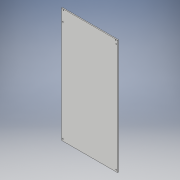
# Autodesk Inventor part: GlyphPlateUnderside
Saved by Autodesk Inventor 2017 (Build 210142000, 142)
## iProperties
Created: 2018-01-27
Part Number: GlyphPlateUnderside
Material: Generic
Document SubType Name: Modeling
Designer: User
Density: 1 g/cm^3
Appearance: Default
Author: User
Autodesk Inventor part; units mm, degrees
ref_plane "YZ Plane" through (0, 0, 0) normal (1, 0, 0) x (0, 1, 0)
ref_plane "XZ Plane" through (0, 0, 0) normal (0, 1, 0) x (-1, 0, 0)
ref_plane "XY Plane" through (0, 0, 0) normal (0, 0, 1) x (1, 0, 0)
sketch "Sketch1" plane through (0, 0, 0) normal (0, 0, 1) x (1, 0, 0)
  line L0 (0, 0) -> (185.8518, 0)
  line L1 (185.8518, 0) -> (185.8518, 381)
  line L2 (185.8518, 381) -> (0, 381)
  line L3 (0, 381) -> (0, 0)
  dimension "d0" = 185.8518
  dimension "d1" = 381
  constraints: 8 end point, 2 parallel, 1 horizontal, 1 perpendicular
  measures "d0" distance of L2.end L1.end
  measures "d1" distance of L1.end L0.end
extrude "Extrusion1" add sketch "Sketch1" along normal blind 3.175
sketch "Sketch2" plane through (0, 0, 3.175) normal (0, 0, 1) x (1, 0, 0)
  line L0 (0, 0) -> (185.8518, 0) projected
  line L1 (0, 0) -> (4.0386, 0)
  line L2 (4.0386, 0) -> (4.0386, 6.35)
  line L3 (0, 381) -> (0, 0) projected
  line L4 (0, 381) -> (4.0386, 381)
  line L5 (185.8518, 381) -> (0, 381) projected
  line L6 (4.0386, 381) -> (4.0386, 342.9)
  line L7 (4.0386, 381) -> (42.1386, 381) construction
  line L8 (0, 381) -> (0, 377.825)
  line L9 (0, 377.825) -> (6.35, 377.825)
  line L10 (185.8518, 0) -> (185.8518, 381) projected
  line L11 (185.8518, 0) -> (181.8132, 0)
  line L12 (181.8132, 0) -> (181.8132, 6.35)
  line L13 (185.8518, 377.825) -> (179.5018, 377.825)
  point P0 (181.8132, 368.3)
  dimension "d4" = 4.0386
  dimension "d5" = 6.35
  dimension "d6" = 38.1
  dimension "d7" = 90
  dimension "d8" = 3.175
  dimension "d9" = 6.35
  dimension "d10" = 4.0386
  dimension "d11" = 6.35
  dimension "d19" = 4.0386
  constraints: 20 end point, 5 coincident, 5 perpendicular, 5 point on line, 1 horizontal, 1 vertical
  measures "d4" distance of L0.start L1.end
  measures "d5" distance of L1.end L2.end
  measures "d6" distance of L4.end L6.end
  measures "d7" angle of L6 L7
  measures "d8" distance of L3.start L8.end
  measures "d9" distance of L8.end L9.end
  measures "d10" distance of L0.end L11.end
  measures "d11" distance of L13.start L13.end
  measures "d19" distance between parallel lines of L3 L6
hole "Hole1" at (4.0386, 6.35, 3.175) at (4.0386, 342.9, 3.175) at (6.35, 377.825, 3.175) at (181.8132, 6.35, 3.175) at (181.8132, 368.3, 3.175) at (179.5018, 377.825, 3.175) direction (0, 0, -1) diameter 3.556 depth 25.4 tip angle 118
body "Solid1"
